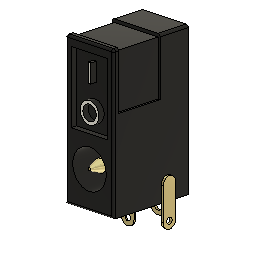
CalendarPrinter Enclosure v23 (Autodesk Fusion 360 archive; units mm, degrees)
design "DC Jack w Rocker Switch"
Autodesk Fusion 360 part; units mm, degrees
sketch "Front Face" plane through (0, 0, 0) normal (0, 1, 0) x (1, 0, 0)
  line L0 (4.5, 12) -> (-4.5, 12)
  line L1 (-4.5, 12) -> (-4.5, -12)
  line L2 (-4.5, -12) -> (4.5, -12)
  line L3 (4.5, -12) -> (4.5, 12)
  line L4 (4.5, 12) -> (-4.5, -12) construction
  line L5 (-4.5, 12) -> (4.5, -12) construction
  circle A0 centre (0, 6) radius 3.15
  line L6 (3.4751, 1) -> (-3.4751, 1)
  line L7 (-3.4751, 1) -> (-3.4751, -10.5)
  line L8 (-3.4751, -10.5) -> (3.4751, -10.5)
  line L9 (3.4751, -10.5) -> (3.4751, 1)
  line L10 (3.4751, 1) -> (-3.4751, -10.5) construction
  line L11 (-3.4751, 1) -> (3.4751, -10.5) construction
  circle A1 centre (0, 6) radius 1.05
  line L12 (0, -12) -> (0, 12) construction
  circle A2 centre (0, -1.9607) radius 1.75
  circle A3 centre (0, -1.9607) radius 1.25
  line L13 (0.25, -6.0814) -> (-0.25, -6.0814)
  line L14 (-0.25, -6.0814) -> (-0.25, -9.0814)
  line L15 (-0.25, -9.0814) -> (0.25, -9.0814)
  line L16 (0.25, -9.0814) -> (0.25, -6.0814)
  line L17 (0.25, -6.0814) -> (-0.25, -9.0814) construction
  line L18 (-0.25, -6.0814) -> (0.25, -9.0814) construction
  point P0 (0, -4.75)
  point P1 (0, -7.5814)
  dimension "d1" = 24
  dimension "d2" = 9
  dimension "d3" = 6.3
  dimension "d4" = 1.5
  dimension "d5" = 1
  dimension "d6" = 6
  dimension "d11" = 2.1
  dimension "d12" = 0.5
  dimension "d13" = 2.5
  dimension "d14" = 0.5
  dimension "d15" = 3
  constraint perpendicular L0 L1
  constraint parallel L0 L2
  constraint parallel L1 L3
  constraint horizontal L0
  constraint coincident L4 origin
  constraint coincident L5 origin
  constraint perpendicular L6 L7
  constraint parallel L6 L8
  constraint parallel L7 L9
  constraint horizontal L6
  constraint coincident L10 P0
  constraint coincident L11 P0
  constraint midpoint L11 P0
  constraint vertical origin P0
  constraint vertical origin A0.centre
  constraint concentric A0 A1
  constraint midpoint L2 L12.start
  constraint midpoint L0 L12.end
  constraint coincident L12 A2.centre
  constraint concentric A2 A3
  constraint perpendicular L13 L14
  constraint parallel L13 L15
  constraint parallel L14 L16
  constraint horizontal L13
  constraint coincident L17 P1
  constraint coincident L18 P1
  constraint coincident L12 P1
  measures "d1" distance of L0.end L1.end
  measures "d2" distance of L1.end L2.end
  measures "d3" diameter of A0
  measures "d4" distance of L2 L8
  measures "d5" distance of origin L6
  measures "d6" distance of L0 A0.centre
  measures "d11" diameter of A1
  measures "d12" distance of A2 A3
  measures "d13" diameter of A3
  measures "d14" distance of L14.end L15.end
  measures "d15" distance of L13.end L14.end
extrude "Extrude1" add sketch "Front Face" along normal blind 14.1 contours L0 L1 L2 L3 | A0 | L6 L7 L8 L9 | A1 | A2 | A3 | L13 L14 L15 L16
extrude "Extrude2" cut sketch "Front Face" along normal blind 10 contours A0
extrude "Extrude3" cut sketch "Front Face" along normal blind 1 contours L6 L7 L8 L9 | A3
chamfer "Chamfer1" distance 0.8 distance2 2 1 edges at (-0.9789, 0, -6.3797) measured on face at (0.3381, 0, -5.6969)
fillet "Fillet1" radius 0.4 6 edges at (4.5, 0, 0) (0, 0, 12) (-4.5, 0, 0) (0, 0, -12) (4.5, 7.05, 12) (-4.5, 7.05, 12)
sketch "Bottom Lugs" plane through (0, 0, -12) normal (0, 0, -1) x (1, 0, 0)
  line L0 (4.5, -0.4) -> (-4.5, -0.4)
  line L1 (-4.5, -0.4) -> (-4.5, -14.1)
  line L2 (-4.5, -14.1) -> (4.5, -14.1)
  line L3 (4.5, -14.1) -> (4.5, -0.4)
  line L4 (-1.2, -7.195) -> (1.2, -7.195)
  line L5 (1.2, -7.195) -> (1.2, -7.445)
  line L6 (1.2, -7.445) -> (-1.2, -7.445)
  line L7 (-1.2, -7.445) -> (-1.2, -7.195)
  line L8 (4.5, -8.985) -> (4.9, -8.985)
  line L9 (4.9, -8.985) -> (4.9, -11.335)
  line L10 (4.9, -11.335) -> (4.5, -11.335)
  line L11 (4.5, -11.335) -> (4.5, -8.985)
  line L12 (-1.65, -13.1) -> (1.2, -13.1)
  line L13 (1.2, -13.1) -> (1.2, -13.5)
  line L14 (1.2, -13.5) -> (-1.65, -13.5)
  line L15 (-1.65, -13.5) -> (-1.65, -13.1)
  line L16 (4.5, 0) -> (-4.5, 0)
  point P0 (0, -7.195)
  point P1 (1.2, -7.32)
  point P2 (1.2, -13.3)
  point P3 (4.7, -11.335)
  point P4 (4.9, -10.16)
  dimension "d21" = 0.25
  dimension "d22" = 2.4
  dimension "d23" = 0.4
  dimension "d24" = 2.35
  dimension "d25" = 2.85
  dimension "d26" = 0.4
  dimension "d28" = 7.32
  dimension "d29" = 13.3
  dimension "d30" = 4.7
  dimension "d33" = 10.16
  constraint horizontal L4
  constraint vertical L5
  constraint horizontal L6
  constraint vertical L7
  constraint horizontal L8
  constraint vertical L9
  constraint horizontal L10
  constraint vertical L11
  constraint horizontal L12
  constraint vertical L13
  constraint horizontal L14
  constraint vertical L15
  constraint collinear L5 L13
  constraint midpoint L4 P0
  constraint vertical origin P0
  constraint midpoint L5 P1
  constraint midpoint L13 P2
  constraint midpoint L10 P3
  constraint midpoint L9 P4
  measures "d21" distance of L4.start L6.end
  measures "d22" distance of L4.start L4.end
  measures "d23" distance of L8.start L8.end
  measures "d24" distance of L8.end L9.end
  measures "d25" distance of L12.start L12.end
  measures "d26" distance of L12.start L14.end
  measures "d28" distance of L16 P1
  measures "d29" distance of L16 P2
  measures "d30" horizontal distance of origin P3
  measures "d33" distance of L16 P4
extrude "Extrude4" add sketch "Bottom Lugs" along normal blind 3.8 contours L4 L5 L6 L7 | L12 L13 L14 L15
extrude "Extrude5" add sketch "Bottom Lugs" along normal mid plane 7.6 contours L3 L8 L9 L10 L11
fillet "Fillet2" radius 1.175 4 edges at (4.7, 8.985, -15.8) (4.7, 11.335, -15.8) (4.7, 8.985, -8.2) (4.7, 11.335, -8.2)
fillet "Fillet2" radius 1.425 2 edges at (1.2, 13.3, -15.8) (-1.65, 13.3, -15.8)
fillet "Fillet2" radius 1.2 2 edges at (1.2, 7.32, -15.8) (-1.2, 7.32, -15.8)
hole "Hole1" at (0, 7.195, -14.6) direction (0, 1, 0) diameter 1 depth 1 tip angle 180
hole "Hole2" at (-0.225, 13.1, -14.375) direction (0, 1, 0) diameter 1.5 depth 1.5 tip angle 180
hole "Hole3" at (4.9, 10.16, -14.625) direction (-1, 0, 0) diameter 1 depth 1 tip angle 180
sketch "Sketch3" plane through (0, 0, 12) normal (0, 0, 1) x (-1, 0, 0)
  line L0 (4.1, -14.1) -> (4.1, -0.4)
  line L1 (4.1, -0.4) -> (-4.1, -0.4)
  line L2 (-4.1, -0.4) -> (-4.1, -14.1)
  line L3 (-4.1, -14.1) -> (4.1, -14.1)
  line L4 (4.5, -0.4) -> (4.5, -14.1)
  line L5 (-4.5, -14.1) -> (-4.5, -0.4)
  line L6 (4.5, -8.8) -> (-4.5, -8.8)
  line L7 (-4.5, -8.8) -> (-4.5, -1)
  line L8 (-4.5, -1) -> (4.5, -1)
  line L9 (4.5, -1) -> (4.5, -8.8)
  line L10 (-4.5, 0) -> (4.5, 0)
  dimension "d48" = 1
  dimension "d49" = 8.8
  constraint horizontal L6
  constraint vertical L7
  constraint horizontal L8
  constraint vertical L9
  constraint coincident L5 L7.end
  constraint coincident L4 L6.start
  measures "d48" distance of L8 L10
  measures "d49" distance of L6 L10
extrude "Extrude6" cut sketch "Sketch3" against normal blind 0.5 contours L0 L2 L6 L8 | L0 L4 L6 L8 L9 | L2 L5 L6 L7 L8
extrude "Extrude7" cut sketch "Sketch3" against normal blind 9.25 contours L0 L4 L6 L8 L9 | L2 L5 L6 L7 L8
equation "d36 = ( 2.35 / 2 ) * 1 mm"
equation "d37 = ( 2.85 / 2 ) * 1 mm"
equation "d38 = ( 2.4 / 2 ) * 1 mm"
equation "d52 = -18.5 mm / 2"

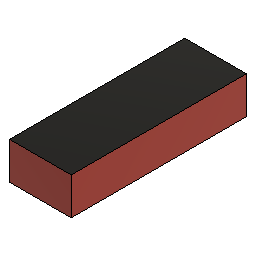
design "5V 3A Power Converter"
Autodesk Fusion 360 part; units mm, degrees
box "BoxPrimitive1" add length 62.5 width 22 height 13.25 placed x (0, 1, 0) y (-1, 0, 0) z (0, 0, 1) at (22, 0, 0)
